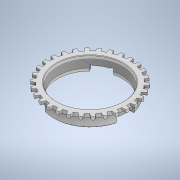
# Autodesk Inventor part: 64. Кольцо блокирующее
Saved by Autodesk Inventor 2021 (Build 250183000, 183)
## iProperties
Created: 2021-03-15
Part Number: 64. Кольцо блокирующее
Material: Типовые
Document SubType Name: Modeling
Designer: Данил
Density: 1 g/cm^3
Appearance: По умолчанию
Author: Данил
Autodesk Inventor part; units mm, degrees
ref_plane "XZ Plane" through (0, 0, 0) normal (0, 1, 0) x (-1, 0, 0)
sketch "Эскиз4" plane through (0, 0, 0) normal (0, 0, 1) x (1, 0, 0)
  line L0 (0, 6.5) -> (0, -6.5)
  line L1 (31.5, -6.5) -> (34.5, -6.5)
  line L2 (35, -6) -> (35, 2.7)
  line L3 (35.3, 3) -> (37, 3)
  line L4 (31.5, -6.5) -> (31.5, -3.5)
  line L5 (31.5, -3.5) -> (30.7735, -3.5)
  line L6 (30.7735, -3.5) -> (31.94, 6)
  line L7 (35, -6) -> (34.5, -6.5)
  arc A0 (35.3, 3) -> (35, 2.7) centre (35.3, 2.7) ccw
  line L8 (37, 3) -> (37, 6.5)
  line L9 (37, 6.5) -> (32.44, 6.5)
  line L10 (31.94, 6) -> (32.44, 6.5)
  point P0 (0, 0)
  point P1 (0, 0)
  point P2 (35, -6.5)
  point P3 (31.94, 6.5)
  dimension "d31" = 13
  dimension "d32" = 63
  dimension "d33" = 70
  dimension "d34" = 3
  dimension "d35" = 7
  dimension "d36" = 0.5
  dimension "d37" = 45
  dimension "d38" = 3.5
  dimension "d39" = 0.3
  dimension "d40" = 74
  dimension "d41" = 0.5
  dimension "d44" = 45
  dimension "d45" = 63.88
  dimension "d46" = 0.5
  constraints: 22 end point, 4 vertical, 3 horizontal, 3 point on line, 2 horizontal alignment, 2 point on circle, 2 tangent, 1 centre point, 1 coincident, 1 midpoint, 1 perpendicular
  measures "d31" distance of L0.start L0.end
  measures "d32" diameter of L1.start L0
  measures "d33" diameter of point (35, -6.5) L0
  measures "d34" distance of L1.start L4.end
  measures "d35" angle of L0 L6
  measures "d36" distance of L2.start point (35, -6.5)
  measures "d37" angle of L2 L7
  measures "d38" distance from line of L0.start L3
  measures "d39" radius of A0
  measures "d40" diameter of L8 L0
  measures "d41" distance of L6.end point (31.94, 6.5)
  measures "d44" angle of L0 L10
  measures "d45" diameter of L6.end L0
  measures "d46" horizontal distance of L9.end L6.end
revolve "Вращение2" add sketch "Эскиз4" angle 360 about axis through (0, 6.5, 0) along (0, -1, 0)
ref_plane "РабПлоскость2" through (35, 0, 0) normal (1, 0, 0) x (0, 1, 0)
sketch "Эскиз5" plane through (35, 0, 0) normal (1, 0, 0) x (0, 1, 0)
  line L0 (-1.5, -8.5) -> (-6.5, -8.5)
  line L1 (-6.5, -8.5) -> (-6.5, 8.5)
  line L2 (-6.5, 8.5) -> (-1.5, 8.5)
  line L3 (-1.5, 8.5) -> (-1.5, -8.5)
  line L4 (-1, 6.5) -> (-6.5, 6.5)
  line L5 (-6.5, 6.5) -> (-6.5, 8.5)
  line L6 (-6.5, 8.5) -> (-1, 8.5)
  line L7 (-1, 8.5) -> (-1, 6.5)
  line L8 (-1, -6.5) -> (-6.5, -6.5)
  line L9 (-6.5, -6.5) -> (-6.5, -8.5)
  line L10 (-6.5, -8.5) -> (-1, -8.5)
  line L11 (-1, -8.5) -> (-1, -6.5)
  line L12 (-6.5, 34.5) -> (-6.5, -34.5) projected
  point P0 (0, 0)
  point P1 (-1.5, 0)
  point P2 (-6.5, 0)
  point P3 (-1.5, -6.5)
  point P4 (-1.5, 6.5)
  dimension "d49" = 17
  dimension "d50" = 2
  dimension "d51" = 5
  dimension "d52" = 0.5
  constraints: 24 end point, 6 parallel, 3 horizontal, 3 midpoint, 3 perpendicular, 1 collinear, 1 horizontal alignment, 1 point on line
  measures "d49" distance of L0.end L1.end
  measures "d50" distance of L6.end L4.start
  measures "d51" distance of L0.start L0.end
  measures "d52" distance between parallel lines of L3 L11
extrude "Выдавливание2" cut sketch "Эскиз5" against normal up to surface round surface about axis through (0, 1.25, 0) along (0, -1, 0) radius 31.3568 half angle -7 far side no
pattern_circular "Круговой массив2" count 3 over 360 about axis through (0, 1.25, 0) along (0, -1, 0) of "Выдавливание2"
thread "Резьба1" size "Rc 1/16" standard "ISO Taper Internal" length 7.4
sketch "Эскиз6" plane through (0, 6.5, 0) normal (0, 1, 0) x (1, 0, 0)
  circle A0 centre (0, 0) radius 40.5 construction
  arc A1 (1.5, 40.4722) -> (-1.5, 40.4722) centre (0, 0) ccw
  circle A2 centre (0, 0) radius 37 projected
  line L0 (-1.5, 40.4722) -> (-2.042, 36.9436)
  circle A3 centre (0, 0) radius 37 projected
  line L1 (1.5, 40.4722) -> (2.042, 36.9436)
  line L2 (-2.042, 36.9436) -> (2.042, 36.9436) construction
  point P0 (0, 40.5)
  point P1 (0, 36.9436)
  dimension "d60" = 81
  dimension "d61" = 4.084
  dimension "d62" = 3
  constraints: 7 point on circle, 6 end point, 2 centre point, 2 coincident, 2 vertical alignment, 1 concentric, 1 horizontal, 1 midpoint
  measures "d60" diameter of A0
  measures "d61" distance of L0.end L1.end
  measures "d62" distance of L0.start L1.start
extrude "Выдавливание3" add sketch "Эскиз6" against normal up to surface (3.5 mm away) contours L1 A2 L0 A1
ref_plane "РабПлоскость3" through (0, 0, -42) normal (0, 0, 1) x (1, 0, 0)
sketch "Эскиз9" plane through (0, 0, -42) normal (0, 0, 1) x (1, 0, 0)
  line L0 (-37, 3) -> (37, 3) projected
  line L1 (-37, 6.5) -> (37, 6.5) projected
  line L2 (-35.3, 3) -> (35.3, 3) projected
  line L3 (0, 3) -> (4.5613, 6.5)
  line L4 (-32.44, 6.5) -> (32.44, 6.5) projected
  line L5 (4.5613, 6.5) -> (4.5613, 3)
  line L6 (0, 3) -> (-4.5613, 6.5)
  line L7 (-4.5613, 6.5) -> (-4.5613, 3)
  point P0 (0, 0)
  point P1 (2.042, 3)
  point P2 (-2.042, 3)
  point P3 (2.042, 6.5)
  point P4 (-2.042, 6.5)
  dimension "d70" = 105
  dimension "d71" = 37.5
  constraints: 8 end point, 4 point on line, 2 perpendicular, 1 midpoint
  measures "d70" angle of L3 L6
  measures "d71" angle of L0 L6
extrude "Выдавливание4" cut sketch "Эскиз9" along normal up to surface contours L7 L6 L0 | L3 L5 L0 round surface about axis through (0, 4.75, 0) along (0, -1, 0) radius 37 far side no
fillet "Сопряжение1" radius 0.4 1 edges at (0, 3, -38.75)
pattern_circular "Круговой массив3" count 30 over 360 about axis through (0, 4.75, 0) along (0, -1, 0) of "Выдавливание3", "Выдавливание4", "Сопряжение1"
